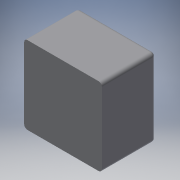
# Autodesk Inventor part: baseFoot
Saved by Autodesk Inventor 2019 (Build 230136000, 136)
## iProperties
Created: 2019-05-07
Part Number: baseFoot
Material: Generic
Document SubType Name: Modeling
Designer: Alex Jones
Density: 1 g/cm^3
Appearance: Default
Author: Alex Jones
Autodesk Inventor part; units mm, degrees
ref_plane "YZ Plane" through (0, 0, 0) normal (1, 0, 0) x (0, 1, 0)
ref_plane "XZ Plane" through (0, 0, 0) normal (0, 1, 0) x (-1, 0, 0)
ref_plane "XY Plane" through (0, 0, 0) normal (0, 0, 1) x (1, 0, 0)
sketch "Sketch1" plane through (0, 0, 0) normal (0, 0, 1) x (1, 0, 0)
  arc A0 (-10, -8.75) -> (-8.75, -10) centre (-8.75, -8.75) ccw projected
  line L0 (-8.75, -10) -> (-3.6, -10) projected
  line L1 (-3.6, -10) -> (-3.1, -9.5) projected
  line L2 (-3.1, -9.5) -> (-3.1, -8.4) projected
  line L3 (-3.1, -8.4) -> (-5.5, -8.4) projected
  line L4 (-5.5, -8.4) -> (-5.5, -6.466) projected
  line L5 (-5.5, -6.466) -> (-3.134, -4.1) projected
  line L6 (-3.134, -4.1) -> (3.134, -4.1) projected
  line L7 (3.134, -4.1) -> (5.5, -6.466) projected
  line L8 (5.5, -6.466) -> (5.5, -8.4) projected
  line L9 (5.5, -8.4) -> (3.1, -8.4) projected
  line L10 (3.1, -8.4) -> (3.1, -9.5) projected
  line L11 (3.1, -9.5) -> (3.6, -10) projected
  line L12 (3.6, -10) -> (8.75, -10) projected
  arc A1 (8.75, -10) -> (10, -8.75) centre (8.75, -8.75) ccw projected
  line L13 (10, -8.75) -> (10, -3.6) projected
  line L14 (10, -3.6) -> (9.5, -3.1) projected
  line L15 (9.5, -3.1) -> (8.4, -3.1) projected
  line L16 (8.4, -3.1) -> (8.4, -5.5) projected
  line L17 (8.4, -5.5) -> (6.466, -5.5) projected
  line L18 (6.466, -5.5) -> (4.1, -3.134) projected
  line L19 (4.1, -3.134) -> (4.1, 3.134) projected
  line L20 (4.1, 3.134) -> (6.466, 5.5) projected
  line L21 (6.466, 5.5) -> (8.4, 5.5) projected
  line L22 (8.4, 5.5) -> (8.4, 3.1) projected
  line L23 (8.4, 3.1) -> (9.5, 3.1) projected
  line L24 (9.5, 3.1) -> (10, 3.6) projected
  line L25 (10, 3.6) -> (10, 8.75) projected
  arc A2 (10, 8.75) -> (8.75, 10) centre (8.75, 8.75) ccw projected
  line L26 (8.75, 10) -> (3.6, 10) projected
  line L27 (3.6, 10) -> (3.1, 9.5) projected
  line L28 (3.1, 9.5) -> (3.1, 8.4) projected
  line L29 (3.1, 8.4) -> (5.5, 8.4) projected
  line L30 (5.5, 8.4) -> (5.5, 6.466) projected
  line L31 (5.5, 6.466) -> (3.134, 4.1) projected
  line L32 (3.134, 4.1) -> (-3.134, 4.1) projected
  line L33 (-3.134, 4.1) -> (-5.5, 6.466) projected
  line L34 (-5.5, 6.466) -> (-5.5, 8.4) projected
  line L35 (-5.5, 8.4) -> (-3.1, 8.4) projected
  line L36 (-3.1, 8.4) -> (-3.1, 9.5) projected
  line L37 (-3.1, 9.5) -> (-3.6, 10) projected
  line L38 (-3.6, 10) -> (-8.75, 10) projected
  arc A3 (-8.75, 10) -> (-10, 8.75) centre (-8.75, 8.75) ccw projected
  line L39 (-10, 8.75) -> (-10, 3.6) projected
  line L40 (-10, 3.6) -> (-9.5, 3.1) projected
  line L41 (-9.5, 3.1) -> (-8.4, 3.1) projected
  line L42 (-8.4, 3.1) -> (-8.4, 5.5) projected
  line L43 (-8.4, 5.5) -> (-6.466, 5.5) projected
  line L44 (-6.466, 5.5) -> (-4.1, 3.134) projected
  line L45 (-4.1, 3.134) -> (-4.1, -3.134) projected
  line L46 (-4.1, -3.134) -> (-6.466, -5.5) projected
  line L47 (-6.466, -5.5) -> (-8.4, -5.5) projected
  line L48 (-8.4, -5.5) -> (-8.4, -3.1) projected
  line L49 (-8.4, -3.1) -> (-9.5, -3.1) projected
  line L50 (-9.5, -3.1) -> (-10, -3.6) projected
  line L51 (-10, -3.6) -> (-10, -8.75) projected
  circle A4 centre (0, 0) radius 2.5 projected
  line L52 (10, 10) -> (-10, 10)
  line L53 (-10, 10) -> (-10, -10)
  line L54 (-10, -10) -> (10, -10)
  line L55 (10, -10) -> (10, 10)
  line L56 (10, 10) -> (-10, -10) construction
  line L57 (-10, 10) -> (10, -10) construction
  line L58 (-10.9523, -10.9523) -> (-10.9523, 10.9523)
  line L59 (-10.9523, 10.9523) -> (10.9523, 10.9523)
  line L60 (10.9523, 10.9523) -> (10.9523, -10.9523)
  line L61 (10.9523, -10.9523) -> (-10.9523, -10.9523)
  line L62 (-13.7358, 13.7358) -> (-13.7358, -13.7358)
  line L63 (-13.7358, -13.7358) -> (13.7358, -13.7358)
  line L64 (13.7358, -13.7358) -> (13.7358, 13.7358)
  line L65 (13.7358, 13.7358) -> (-13.7358, 13.7358)
  constraints: 28 end point, 6 parallel, 3 perpendicular, 2 midpoint, 1 horizontal, 6 other
extrude "Extrusion1" add sketch "Sketch1" against normal blind 12.7 contours L65 L64 L63 L62
sketch "Sketch2" plane through (0, 0, 0) normal (0, 0, 1) x (1, 0, 0)
  line L0 (-13.7358, -13.7358) -> (-13.7358, 13.7358) projected
  line L1 (13.7358, -13.7358) -> (-13.7358, -13.7358)
  line L2 (-13.7358, -13.7358) -> (-13.7358, 13.7358)
  line L3 (-13.7358, 13.7358) -> (13.7358, 13.7358)
  line L4 (13.7358, 13.7358) -> (13.7358, -13.7358)
  line L5 (13.7358, -13.7358) -> (-13.7358, 13.7358) construction
  line L6 (-13.7358, -13.7358) -> (13.7358, 13.7358) construction
  point P0 (0, 0)
  constraints: 12 end point, 2 midpoint, 2 parallel, 1 horizontal, 1 perpendicular
extrude "Extrusion2" add sketch "Sketch2" along normal blind 6.35
fillet "Fillet1" radius 1.1906 12 edges at (13.7358, -13.7358, -3.175) (13.7358, 0, -12.7) (10.9523, 0, -12.7) (0, -13.7358, -12.7) (-13.7358, 0, -12.7) (-13.7358, -13.7358, -3.175) (0, 13.7358, -12.7) (-13.7358, 13.7358, -3.175) (0, -10.9523, -12.7) (-10.9523, 0, -12.7) (0, 10.9523, -12.7) (13.7358, 13.7358, -3.175)
body "Solid1"
